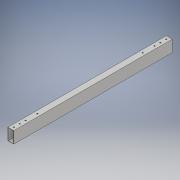
# Autodesk Inventor part: 1x1 27in
Saved by Autodesk Inventor 2018 (Build 220112000, 112)
## iProperties
Created: 2019-01-13
Part Number: 1x1 27in
Material: Generic
Document SubType Name: Modeling
Designer: s-2512711
Density: 1 g/cm^3
Appearance: Default
Author: s-2512711
Autodesk Inventor part; units mm, degrees
ref_plane "YZ Plane" through (0, 0, 0) normal (1, 0, 0) x (0, 1, 0)
ref_plane "XZ Plane" through (0, 0, 0) normal (0, 1, 0) x (-1, 0, 0)
ref_plane "XY Plane" through (0, 0, 0) normal (0, 0, 1) x (1, 0, 0)
sketch "Sketch1" plane through (0, 0, 0) normal (0, 0, 1) x (1, 0, 0)
  line L0 (0, 0) -> (25.4, 0)
  line L1 (25.4, 0) -> (25.4, 50.8)
  line L2 (25.4, 50.8) -> (0, 50.8)
  line L3 (0, 50.8) -> (0, 0)
  line L4 (1.5875, 1.5875) -> (23.8125, 1.5875)
  line L5 (23.8125, 1.5875) -> (23.8125, 49.2125)
  line L6 (23.8125, 49.2125) -> (1.5875, 49.2125)
  line L7 (1.5875, 49.2125) -> (1.5875, 1.5875)
  dimension "d0" = 25.4
  dimension "d1" = 50.8
  dimension "d2" = 1.5875
  constraints: 16 end point, 4 parallel, 2 perpendicular, 1 horizontal, 3 other
  measures "d0" distance of L2.end L1.end
  measures "d1" distance of L1.end L0.end
  measures "d2" distance between parallel lines of L3 L7
extrude "Extrusion1" add sketch "Sketch1" along normal blind 685.8
sketch "Sketch2" plane through (0, 50.8, 0) normal (0, 1, 0) x (1, 0, 0)
  line L0 (25.4, 0) -> (0, 0) construction
  line L1 (12.7, 0) -> (12.7, -12.7) construction
  line L2 (12.7, -12.7) -> (12.7, -38.1) construction
  line L3 (0, 0) -> (0, -685.8) construction
  line L4 (0, -342.9) -> (25.4, -342.9) construction
  circle A0 centre (12.7, -38.1) radius 2.5797
  circle A1 centre (12.7, -12.7) radius 2.5797
  line L5 (25.4, -685.8) -> (0, -685.8) construction
  line L6 (12.7, -685.8) -> (12.7, -673.1) construction
  line L7 (12.7, -673.1) -> (12.7, -647.7) construction
  line L8 (0, -685.8) -> (0, 0) construction
  circle A2 centre (12.7, -647.7) radius 2.5797
  circle A3 centre (12.7, -673.1) radius 2.5797
  dimension "d5" = 12.7
  dimension "d6" = 25.4
  dimension "d7" = 5.1594
  constraints: 14 end point, 8 symmetric about line, 4 centre point, 4 coincident, 2 midpoint, 2 point on line, 1 horizontal, 1 vertical, 2 other
  measures "d5" distance of L1.start L1.end
  measures "d6" distance of L1.end L2.end
  measures "d7" diameter of A0
extrude "Extrusion2" cut sketch "Sketch2" against normal blind 165.1
sketch "Sketch5" plane through (0, 50.8, 0) normal (0, 1, 0) x (1, 0, 0)
  circle A0 centre (12.7, -38.1) radius 2.5797 construction
  line L0 (12.7, -38.1) -> (12.7, -63.5) construction
  line L1 (0, 0) -> (0, -685.8) construction
  line L2 (0, -342.9) -> (25.4, -342.9) construction
  line L3 (25.4, 0) -> (25.4, -685.8) construction
  circle A1 centre (12.7, -63.5) radius 2.5797
  line L4 (12.7, -63.5) -> (12.7, -114.3) construction
  circle A2 centre (12.7, -114.3) radius 2.5797
  circle A3 centre (12.7, -622.3) radius 2.5797
  circle A4 centre (12.7, -571.5) radius 2.5797
  dimension "d27" = 25.4
  dimension "d29" = 50.8
  constraints: 6 end point, 4 centre point, 2 coincident, 2 midpoint, 2 symmetric about line, 2 vertical, 2 other
  measures "d27" distance of L0.start L0.end
  measures "d29" distance of L4.start L4.end
extrude "Extrusion8" cut sketch "Sketch5" against normal blind 331.7875
body "Solid1"
